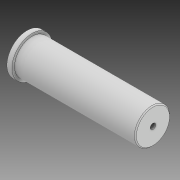
# Autodesk Inventor part: J1_pin
Saved by Autodesk Inventor 2020 (Build 240168000, 168)
## iProperties
Created: 2021-03-26
Part Number: J1_pin
Material: Generic
Document SubType Name: Modeling
Designer: DDeGo
Density: 1 g/cm^3
Appearance: Default
Author: DDeGo
Autodesk Inventor part; units mm, degrees
ref_plane "YZ Plane" through (0, 0, 0) normal (1, 0, 0) x (0, 1, 0)
ref_plane "XZ Plane" through (0, 0, 0) normal (0, 1, 0) x (-1, 0, 0)
ref_plane "XY Plane" through (0, 0, 0) normal (0, 0, 1) x (1, 0, 0)
sketch "Sketch1" plane through (0, 0, 0) normal (0, 0, 1) x (1, 0, 0)
  line L0 (0, 0) -> (0, 4.5) construction
  line L1 (0, 4.5) -> (0, 19.9)
  line L2 (0, 19.9) -> (5, 19.9)
  line L3 (5, 19.9) -> (5, 17.4)
  line L4 (5, 17.4) -> (124.5, 17.4)
  line L5 (124.5, 17.4) -> (124.5, 2.7)
  line L6 (124.5, 2.7) -> (109.5, 2.7)
  line L7 (109.5, 2.7) -> (109.5, 4.5)
  line L8 (109.5, 4.5) -> (0, 4.5)
  line L9 (0, 0) -> (13.4104, 0) construction
  dimension "d0" = 2.7
  dimension "d1" = 4.5
  dimension "d2" = 15
  dimension "d3" = 5
  dimension "d4" = 17.4
  dimension "d5" = 2.5
  dimension "d6" = 119.5
  constraints: 21 end point, 7 perpendicular, 1 horizontal, 1 point on line, 1 vertical
  measures "d0" distance between parallel lines of L9 L6
  measures "d1" distance between parallel lines of L9 L8
  measures "d2" distance between parallel lines of L5 L7
  measures "d3" distance between parallel lines of L1 L3
  measures "d4" distance between parallel lines of L9 L4
  measures "d5" distance between parallel lines of L4 L2
  measures "d6" distance between parallel lines of L5 L3
revolve "Revolution1" add sketch "Sketch1" angle 360 about axis through (0, 0, 0) along (1, 0, 0)
chamfer "Chamfer1" distance 1 angle 45 1 edges at (124.5, -17.4, 0)
body "Solid1"
